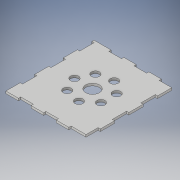
# Autodesk Inventor part: KIRI
Saved by Autodesk Inventor 2019 (Build 230136000, 136)
## iProperties
Created: 2019-11-24
Part Number: KIRI
Material: Generic
Document SubType Name: Modeling
Designer: User
Density: 1 g/cm^3
Appearance: Default
Author: User
Autodesk Inventor part; units mm, degrees
ref_plane "YZ Plane" through (0, 0, 0) normal (1, 0, 0) x (0, 1, 0)
ref_plane "XZ Plane" through (0, 0, 0) normal (0, 1, 0) x (-1, 0, 0)
ref_plane "XY Plane" through (0, 0, 0) normal (0, 0, 1) x (1, 0, 0)
sketch "Sketch1" plane through (0, 0, 0) normal (0, 1, 0) x (-1, 0, 0)
  line L0 (34, 37.5) -> (-34, -37.5) construction
  line L1 (-34, 37.5) -> (34, -37.5) construction
  line L2 (34, 37.5) -> (34, 25)
  line L3 (34, 25) -> (32, 25)
  line L4 (32, 25) -> (32, 12.5)
  line L5 (32, 12.5) -> (34, 12.5)
  line L6 (34, 12.5) -> (34, 0)
  line L7 (34, 0) -> (32, 0)
  line L8 (32, 0) -> (32, -12.5)
  line L9 (32, -12.5) -> (34, -12.5)
  line L10 (34, -12.5) -> (34, -25)
  line L11 (34, -25) -> (32, -25)
  line L12 (32, -25) -> (32, -37.5)
  line L13 (34, -25) -> (34, -12.5)
  line L14 (34, 0) -> (34, 12.5)
  line L15 (34, 25) -> (34, 37.5)
  line L16 (-3, -37.5) -> (-14, -37.5)
  line L17 (-14, -37.5) -> (-14, -39.5)
  line L18 (-14, -39.5) -> (-25, -39.5)
  line L19 (-25, -39.5) -> (-25, -37.5)
  line L20 (-34, -37.5) -> (-36, -37.5)
  line L21 (-36, -37.5) -> (-36, -25)
  line L22 (-36, -25) -> (-34, -25)
  line L23 (-34, -25) -> (-34, -12.5)
  line L24 (-34, -12.5) -> (-36, -12.5)
  line L25 (-36, -12.5) -> (-36, 0)
  line L26 (-36, 0) -> (-34, 0)
  line L27 (-34, 0) -> (-34, 12.5)
  line L28 (-34, 12.5) -> (-34, 8.9552)
  line L29 (-34, 12.5) -> (-36, 12.5)
  line L30 (-36, 12.5) -> (-36, 25)
  line L31 (-36, 25) -> (-34, 25)
  line L32 (-34, -37.5) -> (-25, -37.5)
  line L33 (-14, -37.5) -> (-3, -37.5)
  line L34 (-34, -12.5) -> (-34, -25)
  line L35 (-34, 35.5) -> (-34, 25)
  line L36 (-34, 12.5) -> (-34, 0)
  line L37 (34, 37.5) -> (23, 37.5)
  line L38 (23, 37.5) -> (23, 35.5)
  line L39 (23, 35.5) -> (12, 35.5)
  line L40 (12, 35.5) -> (12, 37.5)
  line L41 (12, 37.5) -> (1, 37.5)
  line L42 (1, 37.5) -> (1, 35.5)
  line L43 (1, 35.5) -> (-10, 35.5)
  line L44 (-10, 35.5) -> (-10, 37.5)
  line L45 (-10, 37.5) -> (-21, 37.5)
  line L46 (-21, 37.5) -> (-21, 35.5)
  line L47 (-21, 35.5) -> (-34, 35.5)
  line L48 (34, 37.5) -> (23, 37.5)
  line L49 (12, 37.5) -> (1, 37.5)
  line L50 (-10, 37.5) -> (-21, 37.5)
  circle A0 centre (-2.2106, -2.0043) radius 6
  circle A1 centre (13.57, -2.0043) radius 3.5
  circle A2 centre (7.6284, 10.3335) radius 3.5
  circle A3 centre (-5.7222, 13.3806) radius 3.5
  circle A4 centre (-16.4285, 4.8426) radius 3.5
  circle A5 centre (-16.4285, -8.8513) radius 3.5
  circle A6 centre (-5.7222, -17.3893) radius 3.5
  circle A7 centre (7.6284, -14.3421) radius 3.5
  line L51 (-3, -37.5) -> (-3, -39.5)
  line L52 (-3, -39.5) -> (8, -39.5)
  line L53 (8, -39.5) -> (8, -37.5)
  line L54 (8, -37.5) -> (19, -37.5)
  line L55 (19, -37.5) -> (19, -39.5)
  line L56 (19, -39.5) -> (32, -39.5)
  line L57 (32, -39.5) -> (34, -39.5)
  line L58 (34, -39.5) -> (34, -37.5)
  line L59 (32, -37.5) -> (34, -37.5)
  point P0 (0, 0)
  point P1 (0, 0)
  point P2 (8.5, -39.5)
  point P3 (-2.5, -39.5)
  dimension "d1" = 75
  dimension "d2" = 2
  dimension "d3" = 12.5
  dimension "d4" = 12.5
  dimension "d5" = 12.5
  dimension "d6" = 12.5
  dimension "d7" = 2
  dimension "d13" = 11
  dimension "d14" = 2
  dimension "d15" = 12.5
  dimension "d16" = 12.5
  dimension "d17" = 2
  dimension "d18" = 12.5
  dimension "d19" = 12.5
  dimension "d20" = 2
  dimension "d21" = 12.5
  dimension "d22" = 11
  dimension "d23" = 11
  dimension "d24" = 11
  dimension "d25" = 11
  dimension "d28" = 12
  dimension "d29" = 7
  dimension "d30" = 360
  dimension "d33" = 9
  dimension "d34" = 11
  dimension "d35" = 11
  dimension "d36" = 2
  dimension "d37" = 11
  constraints: 120 end point, 47 perpendicular, 15 parallel, 12 point on line, 8 centre point, 5 horizontal, 2 midpoint, 1 vertical, 15 other
  measures "d1" distance of L1.start L0.end
  measures "d2" distance of L2.end L3.end
  measures "d3" distance of L3.end L4.end
  measures "d4" distance of L5.end L7.start
  measures "d5" distance of L8.start L9.start
  measures "d6" distance of L11.start L10.start
  measures "d7" distance of L11.start L12.start
  measures "d13" distance of L17.end L18.end
  measures "d14" distance of L0.end L20.end
  measures "d15" distance of L20.end L21.end
  measures "d16" distance of L22.end L23.end
  measures "d17" distance of L23.end L24.end
  measures "d18" distance of L24.end L26.start
  measures "d19" distance of L26.end L27.end
  measures "d20" distance of L27.end L30.start
  measures "d21" distance of L30.start L31.start
  measures "d22" distance of L0.start L38.start
  measures "d23" distance of L41.start L42.start
  measures "d24" distance of L43.start L43.end
  measures "d25" distance of L45.end L44.end
  measures "d28" diameter of A0
  measures "d29" diameter of A1
  measures "d33" distance of L0.end L19.end
  measures "d34" distance of L16.end L16.start
  measures "d35" distance of L51.end L52.end
  measures "d36" distance of L52.end L53.end
  measures "d37" distance of L53.end L54.end
extrude "Extrusion1" add sketch "Sketch1" along normal blind 2
body "Solid1"
